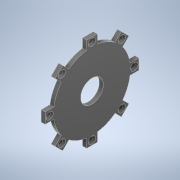
# Autodesk Inventor part: Gear_Box_Chasis_Divider
Saved by Autodesk Inventor 2022 (Build 260153000, 153)
## iProperties
Created: 2022-04-22
Part Number: Gear_Box_Chasis_Divider
Material: ABS Plastic
Document SubType Name: Modeling
Designer: Mlees
Density: 1.06 g/cm^3
Appearance: Smooth - Black
Mass: 8.52567 g
Surface Area: 66.5001 cm^2
Volume: 8.04309 cm^3
Author: Mlees
Autodesk Inventor part; units mm, degrees
ref_plane "YZ Plane" through (0, 0, 0) normal (1, 0, 0) x (0, 1, 0)
ref_plane "XZ Plane" through (0, 0, 0) normal (0, 1, 0) x (-1, 0, 0)
ref_plane "XY Plane" through (0, 0, 0) normal (0, 0, 1) x (1, 0, 0)
sketch "Sketch1" plane through (0, 0, 0) normal (1, 0, 0) x (0, 1, 0)
  circle A0 centre (0, 0) radius 8.5
  line L0 (28.3441, -4) -> (35, -4)
  line L1 (35, 4) -> (35, -4)
  line L2 (28.3441, 4) -> (35, 4)
  circle A1 centre (31.6721, 0) radius 1.625
  line L3 (17.2139, 22.8708) -> (21.9203, 27.5772)
  line L4 (21.9203, 27.5772) -> (27.5772, 21.9203)
  circle A2 centre (22.3955, 22.3955) radius 1.625
  line L5 (22.8708, 17.2139) -> (27.5772, 21.9203)
  line L6 (-4, 28.3441) -> (-4, 35)
  line L7 (-4, 35) -> (4, 35)
  circle A3 centre (0, 31.6721) radius 1.625
  line L8 (4, 28.3441) -> (4, 35)
  line L9 (-22.8708, 17.2139) -> (-27.5772, 21.9203)
  line L10 (-27.5772, 21.9203) -> (-21.9203, 27.5772)
  circle A4 centre (-22.3955, 22.3955) radius 1.625
  line L11 (-17.2139, 22.8708) -> (-21.9203, 27.5772)
  line L12 (-28.3441, -4) -> (-35, -4)
  line L13 (-35, -4) -> (-35, 4)
  circle A5 centre (-31.6721, 0) radius 1.625
  line L14 (-28.3441, 4) -> (-35, 4)
  line L15 (-17.2139, -22.8708) -> (-21.9203, -27.5772)
  line L16 (-21.9203, -27.5772) -> (-27.5772, -21.9203)
  circle A6 centre (-22.3955, -22.3955) radius 1.625
  line L17 (-22.8708, -17.2139) -> (-27.5772, -21.9203)
  line L18 (4, -28.3441) -> (4, -35)
  line L19 (4, -35) -> (-4, -35)
  circle A7 centre (0, -31.6721) radius 1.625
  line L20 (-4, -28.3441) -> (-4, -35)
  line L21 (22.8708, -17.2139) -> (27.5772, -21.9203)
  line L22 (27.5772, -21.9203) -> (21.9203, -27.5772)
  circle A8 centre (22.3955, -22.3955) radius 1.625
  line L23 (17.2139, -22.8708) -> (21.9203, -27.5772)
  arc A9 (22.8708, -17.2139) -> (28.3441, -4) centre (0, 0) ccw
  arc A10 (4, -28.3441) -> (17.2139, -22.8708) centre (0, 0) ccw
  arc A11 (-17.2139, -22.8708) -> (-4, -28.3441) centre (0, 0) ccw
  arc A12 (-28.3441, -4) -> (-22.8708, -17.2139) centre (0, 0) ccw
  arc A13 (-22.8708, 17.2139) -> (-28.3441, 4) centre (0, 0) ccw
  arc A14 (-4, 28.3441) -> (-17.2139, 22.8708) centre (0, 0) ccw
  arc A15 (28.3441, 4) -> (22.8708, 17.2139) centre (0, 0) ccw
  arc A16 (17.2139, 22.8708) -> (4, 28.3441) centre (0, 0) ccw
  dimension "d0" = 17
  dimension "d8" = 360
  dimension "d12" = 3.25
  constraints: 48 end point, 17 centre point, 16 point on circle, 2 coincident, 1 vertical, 73 other
  measures "d0" diameter of A0
  measures "d12" diameter of A1
extrude "Extrusion1" add sketch "Sketch1" along normal blind 3
sketch "Sketch2" plane through (3, 0, 0) normal (1, 0, 0) x (0, 0, -1)
  line L0 (-5.2542, 23.7941) -> (-5.2542, 26.8421)
  line L1 (-5.2542, 26.8421) -> (-2.9174, 26.8421)
  line L2 (-2.9174, 26.8421) -> (-2.9174, 26.5373)
  line L3 (-2.9174, 26.5373) -> (-4.9494, 26.5373)
  line L4 (-4.9494, 26.5373) -> (-4.9494, 25.5721)
  line L5 (-4.9494, 25.5721) -> (-2.9174, 25.5721)
  line L6 (-2.9174, 25.5721) -> (-2.9174, 25.2673)
  line L7 (-2.9174, 25.2673) -> (-4.9494, 25.2673)
  line L8 (-4.9494, 25.2673) -> (-4.9494, 23.7941)
  line L9 (-4.9494, 23.7941) -> (-5.2542, 23.7941)
  line L10 (-5.2034, 23.8449) -> (-5.2034, 26.7913)
  line L11 (-5.2034, 26.7913) -> (-2.9682, 26.7913)
  line L12 (-2.9682, 26.7913) -> (-2.9682, 26.5881)
  line L13 (-2.9682, 26.5881) -> (-5.0002, 26.5881)
  line L14 (-5.0002, 26.5881) -> (-5.0002, 25.5213)
  line L15 (-5.0002, 25.5213) -> (-2.9682, 25.5213)
  line L16 (-2.9682, 25.5213) -> (-2.9682, 25.3181)
  line L17 (-2.9682, 25.3181) -> (-5.0002, 25.3181)
  line L18 (-5.0002, 25.3181) -> (-5.0002, 23.8449)
  line L19 (-5.0002, 23.8449) -> (-5.2034, 23.8449)
  line L20 (-5.1526, 23.8957) -> (-5.1526, 26.7405)
  line L21 (-5.1526, 26.7405) -> (-3.019, 26.7405)
  line L22 (-3.019, 26.7405) -> (-3.019, 26.6389)
  line L23 (-3.019, 26.6389) -> (-5.051, 26.6389)
  line L24 (-5.051, 26.6389) -> (-5.051, 25.4705)
  line L25 (-5.051, 25.4705) -> (-3.019, 25.4705)
  line L26 (-3.019, 25.4705) -> (-3.019, 25.3689)
  line L27 (-3.019, 25.3689) -> (-5.051, 25.3689)
  line L28 (-5.051, 25.3689) -> (-5.051, 23.8957)
  line L29 (-5.051, 23.8957) -> (-5.1526, 23.8957)
  line L30 (-5.1018, 23.9465) -> (-5.1018, 26.6897)
  line L31 (-5.1018, 26.6897) -> (-3.0698, 26.6897)
  line L32 (-3.0698, 25.4197) -> (-5.1018, 25.4197)
  line L33 (-2.511, 23.7941) -> (-2.511, 26.0293)
  line L34 (-2.511, 26.0293) -> (-2.2062, 26.0293)
  line L35 (-2.2062, 26.0293) -> (-2.2062, 25.6737)
  arc A0 (-1.3889, 26.0291) -> (-2.2062, 25.6737) centre (-1.3889, 24.9115) ccw
  line L36 (-1.3889, 26.0291) -> (-1.0841, 26.0291)
  line L37 (-1.0841, 26.0291) -> (-1.0841, 25.7243)
  line L38 (-1.0841, 25.7243) -> (-1.3889, 25.7243)
  arc A1 (-1.3889, 25.7243) -> (-2.2017, 24.9115) centre (-1.3889, 24.9115) ccw
  line L39 (-2.2017, 24.9115) -> (-2.2017, 23.7939)
  line L40 (-2.2017, 23.7939) -> (-2.5065, 23.7939)
  line L41 (-2.4557, 23.8447) -> (-2.4557, 24.9115)
  arc A2 (-1.3889, 25.9783) -> (-2.4557, 24.9115) centre (-1.3889, 24.9115) ccw
  line L42 (-1.3889, 25.9783) -> (-1.1349, 25.9783)
  line L43 (-1.1349, 25.9783) -> (-1.1349, 25.7751)
  line L44 (-1.1349, 25.7751) -> (-1.3889, 25.7751)
  arc A3 (-1.3889, 25.7751) -> (-2.2525, 24.9115) centre (-1.3889, 24.9115) ccw
  line L45 (-2.2525, 24.9115) -> (-2.2525, 23.8447)
  line L46 (-2.2525, 23.8447) -> (-2.4557, 23.8447)
  line L47 (-2.4049, 23.8955) -> (-2.4049, 24.9115)
  arc A4 (-1.3889, 25.9275) -> (-2.4049, 24.9115) centre (-1.3889, 24.9115) ccw
  line L48 (-1.3889, 25.9275) -> (-1.1857, 25.9275)
  line L49 (-1.1857, 25.9275) -> (-1.1857, 25.8259)
  line L50 (-1.1857, 25.8259) -> (-1.3889, 25.8259)
  arc A5 (-1.3889, 25.8259) -> (-2.3033, 24.9115) centre (-1.3889, 24.9115) ccw
  line L51 (-2.3033, 24.9115) -> (-2.3033, 23.8955)
  line L52 (-2.3033, 23.8955) -> (-2.4049, 23.8955)
  line L53 (-2.3541, 23.9463) -> (-2.3541, 24.9115)
  arc A6 (-1.3889, 25.8767) -> (-2.3541, 24.9115) centre (-1.3889, 24.9115) ccw
  line L54 (-1.3889, 25.8767) -> (-1.2365, 25.8767)
  line L55 (-2.4557, 24.9115) -> (-2.4557, 25.9783)
  line L56 (-2.4557, 25.9783) -> (-2.2525, 25.9783)
  line L57 (-2.2525, 25.9783) -> (-2.2525, 25.5211)
  line L58 (-2.3033, 25.4703) -> (-2.3033, 25.9275)
  line L59 (-2.3033, 25.9275) -> (-2.4049, 25.9275)
  line L60 (-2.4049, 25.9275) -> (-2.4049, 25.2163)
  line L61 (-2.3541, 25.3687) -> (-2.3541, 25.8767)
  circle A7 centre (0.4399, 24.9115) radius 1.1176
  circle A8 centre (0.4399, 24.9115) radius 0.8128
  circle A9 centre (0.4399, 24.9115) radius 0.8636
  circle A10 centre (0.4399, 24.9115) radius 0.9144
  circle A11 centre (0.4399, 24.9115) radius 0.9652
  circle A12 centre (0.4399, 24.9115) radius 1.016
  circle A13 centre (0.4399, 24.9115) radius 1.0668
  line L62 (1.9639, 23.7939) -> (1.9639, 26.0291)
  line L63 (1.9639, 26.0291) -> (2.2687, 26.0291)
  line L64 (2.2687, 26.0291) -> (2.2687, 25.8005)
  arc A14 (3.795, 25.121) -> (2.2687, 25.8005) centre (2.8806, 25.121) ccw
  line L65 (3.795, 25.121) -> (3.795, 23.8002)
  line L66 (3.795, 23.8002) -> (3.4902, 23.8002)
  line L67 (3.4902, 23.8002) -> (3.4902, 25.121)
  arc A15 (3.4902, 25.121) -> (2.271, 25.121) centre (2.8806, 25.121) ccw
  line L68 (2.271, 25.121) -> (2.271, 23.8002)
  line L69 (2.271, 23.8002) -> (1.9662, 23.8002)
  line L70 (2.017, 23.851) -> (2.017, 25.121)
  arc A16 (3.7442, 25.121) -> (2.017, 25.121) centre (2.8806, 25.121) ccw
  line L71 (3.7442, 25.121) -> (3.7442, 23.851)
  line L72 (3.7442, 23.851) -> (3.541, 23.851)
  line L73 (3.541, 23.851) -> (3.541, 25.121)
  arc A17 (3.541, 25.121) -> (2.2202, 25.121) centre (2.8806, 25.121) ccw
  line L74 (2.2202, 25.121) -> (2.2202, 23.851)
  line L75 (2.2202, 23.851) -> (2.017, 23.851)
  line L76 (2.0678, 23.9018) -> (2.0678, 25.121)
  arc A18 (3.6934, 25.121) -> (2.0678, 25.121) centre (2.8806, 25.121) ccw
  line L77 (3.6934, 25.121) -> (3.6934, 23.9018)
  line L78 (3.6934, 23.9018) -> (3.5918, 23.9018)
  line L79 (3.5918, 23.9018) -> (3.5918, 25.121)
  arc A19 (3.5918, 25.121) -> (2.1694, 25.121) centre (2.8806, 25.121) ccw
  line L80 (2.1694, 25.121) -> (2.1694, 23.9018)
  line L81 (2.1694, 23.9018) -> (2.0678, 23.9018)
  line L82 (2.1186, 23.9526) -> (2.1186, 25.121)
  arc A20 (3.6426, 25.121) -> (2.1186, 25.121) centre (2.8806, 25.121) ccw
  line L83 (3.6426, 25.121) -> (3.6426, 23.9526)
  line L84 (2.017, 25.121) -> (2.017, 25.9846)
  line L85 (2.017, 25.9846) -> (2.2202, 25.9846)
  line L86 (2.2202, 25.9846) -> (2.2202, 25.6798)
  line L87 (2.1694, 25.629) -> (2.1694, 25.9338)
  line L88 (2.1694, 25.9338) -> (2.0678, 25.9338)
  line L89 (2.0678, 25.9338) -> (2.0678, 25.375)
  line L90 (2.1186, 25.5274) -> (2.1186, 25.883)
  arc A21 (4.4554, 24.2066) -> (4.8618, 23.8002) centre (4.8618, 24.2066) ccw
  line L91 (4.4554, 24.2066) -> (4.4554, 25.7306)
  line L92 (4.4554, 25.7306) -> (4.1506, 25.7306)
  line L93 (4.1506, 25.7306) -> (4.1506, 26.0354)
  line L94 (4.1506, 26.0354) -> (4.4554, 26.0354)
  line L95 (4.4554, 26.0354) -> (4.4554, 26.8482)
  line L96 (4.4554, 26.8482) -> (4.7602, 26.8482)
  line L97 (4.7602, 26.8482) -> (4.7602, 26.0354)
  line L98 (4.7602, 26.0354) -> (5.065, 26.0354)
  line L99 (5.065, 26.0354) -> (5.065, 25.7306)
  line L100 (5.065, 25.7306) -> (4.7602, 25.7306)
  line L101 (4.7602, 25.7306) -> (4.7602, 24.2066)
  arc A22 (4.7602, 24.2066) -> (4.8618, 24.105) centre (4.8618, 24.2066) ccw
  line L102 (4.8618, 24.105) -> (5.065, 24.105)
  line L103 (5.065, 24.105) -> (5.065, 23.8002)
  line L104 (5.065, 23.8002) -> (4.8618, 23.8002)
  arc A23 (4.5062, 24.2066) -> (4.8618, 23.851) centre (4.8618, 24.2066) ccw
  line L105 (4.5062, 24.2066) -> (4.5062, 25.7814)
  line L106 (4.5062, 25.7814) -> (4.2014, 25.7814)
  line L107 (4.2014, 25.7814) -> (4.2014, 25.9846)
  line L108 (4.2014, 25.9846) -> (4.5062, 25.9846)
  line L109 (4.5062, 25.9846) -> (4.5062, 26.7974)
  line L110 (4.5062, 26.7974) -> (4.7094, 26.7974)
  line L111 (4.7094, 26.7974) -> (4.7094, 25.9846)
  line L112 (4.7094, 25.9846) -> (5.0142, 25.9846)
  line L113 (5.0142, 25.9846) -> (5.0142, 25.7814)
  line L114 (5.0142, 25.7814) -> (4.7094, 25.7814)
  line L115 (4.7094, 25.7814) -> (4.7094, 24.2066)
  arc A24 (4.7094, 24.2066) -> (4.8618, 24.0542) centre (4.8618, 24.2066) ccw
  line L116 (4.8618, 24.0542) -> (5.0142, 24.0542)
  line L117 (5.0142, 24.0542) -> (5.0142, 23.851)
  line L118 (5.0142, 23.851) -> (4.8618, 23.851)
  arc A25 (4.557, 24.2066) -> (4.8618, 23.9018) centre (4.8618, 24.2066) ccw
  line L119 (4.557, 24.2066) -> (4.557, 25.8322)
  line L120 (4.557, 25.8322) -> (4.2522, 25.8322)
  line L121 (4.2522, 25.8322) -> (4.2522, 25.9338)
  line L122 (4.2522, 25.9338) -> (4.557, 25.9338)
  line L123 (4.557, 25.9338) -> (4.557, 26.7466)
  line L124 (4.557, 26.7466) -> (4.6586, 26.7466)
  line L125 (4.6586, 26.7466) -> (4.6586, 25.9338)
  line L126 (4.6586, 25.9338) -> (4.9634, 25.9338)
  line L127 (4.9634, 25.9338) -> (4.9634, 25.8322)
  line L128 (4.9634, 25.8322) -> (4.6586, 25.8322)
  line L129 (4.6586, 25.8322) -> (4.6586, 24.2066)
  arc A26 (4.6586, 24.2066) -> (4.8618, 24.0034) centre (4.8618, 24.2066) ccw
  line L130 (4.8618, 24.0034) -> (4.9634, 24.0034)
  line L131 (4.9634, 24.0034) -> (4.9634, 23.9018)
  line L132 (4.9634, 23.9018) -> (4.8618, 23.9018)
  line L133 (4.9126, 23.9526) -> (4.8618, 23.9526)
  arc A27 (4.6078, 24.2066) -> (4.8618, 23.9526) centre (4.8618, 24.2066) ccw
  line L134 (4.6078, 24.2066) -> (4.6078, 26.6958)
  line L135 (4.303, 25.883) -> (4.9126, 25.883)
  point P0 (0, 0)
  point P1 (-2.2525, 25.5378)
extrude "Extrusion2" [suppressed]
chamfer "Chamfer1" distance 1.1 angle 45 8 edges at (3, 30.0471, 0) (3, 20.7705, -22.3955) (3, -1.625, -31.6721) (3, -24.0205, -22.3955) (3, -33.2971, 0) (3, -24.0205, 22.3955) (3, -1.625, 31.6721) (3, 20.7705, 22.3955)
body "Solid1"
